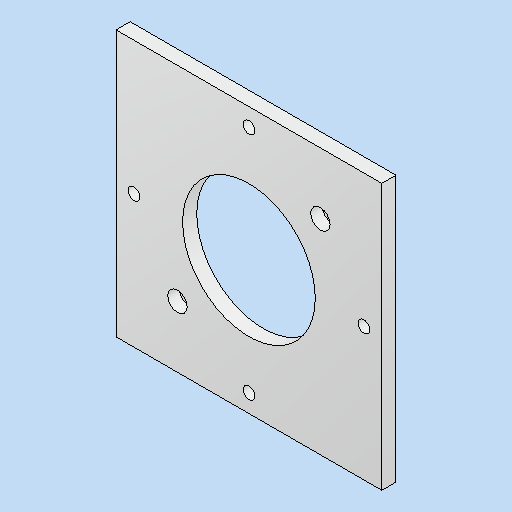
# Autodesk Inventor part: FLI-Al-Plate
Saved by Autodesk Inventor 2025 (Build 290162000, 162)
## iProperties
Created: 2025-02-17
Part Number: FLI-Al-Plate
Material: Aluminum 6061
Document SubType Name: Modeling
Designer: kuzmin
Density: 2.7 g/cm^3
Appearance: Aluminum - Flat
Author: kuzmin
Autodesk Inventor part; units mm, degrees
ref_plane "YZ Plane" through (0, 0, 0) normal (1, 0, 0) x (0, 1, 0)
ref_plane "XZ Plane" through (0, 0, 0) normal (0, 1, 0) x (-1, 0, 0)
ref_plane "XY Plane" through (0, 0, 0) normal (0, 0, 1) x (1, 0, 0)
sketch "Sketch1" plane through (0, 0, 0) normal (0, 0, 1) x (1, 0, 0)
  line L0 (-75.15, 75.15) -> (75.15, 75.15)
  line L1 (75.15, 75.15) -> (75.15, -75.15)
  line L2 (75.15, -75.15) -> (-75.15, -75.15)
  line L3 (-75.15, -75.15) -> (-75.15, 75.15)
  circle A0 centre (40.4112, 40.4112) radius 3.4
  circle A1 centre (-40.4112, -40.4112) radius 3.4
  circle A2 centre (-65, 0) radius 3.35
  circle A3 centre (0, -65) radius 3.35
  circle A4 centre (0, 65) radius 3.35
  circle A5 centre (65, 0) radius 3.35
  circle A6 centre (0, 0) radius 65 construction
  circle A7 centre (0, 0) radius 37.5
  circle A8 centre (0, 0) radius 57.15 construction
  line L4 (40.4112, 40.4112) -> (-40.4112, -40.4112) construction
  point P0 (0, 75.15)
  point P1 (75.15, 0)
  dimension "d14" = 150.3
  dimension "d26" = 6.7
  dimension "d32" = 130
  dimension "d33" = 75
  dimension "d40" = 114.3
  dimension "d42" = 6.8
  dimension "d43" = 45
  constraints: 10 end point, 9 centre point, 6 point on circle, 4 coincident, 4 equal radius, 3 horizontal alignment, 3 midpoint, 3 vertical alignment, 2 parallel, 2 perpendicular, 1 horizontal
  measures "d14" distance of L0.start L0.end
  measures "d26" diameter of A4
  measures "d32" diameter of A6
  measures "d33" diameter of A7
  measures "d40" diameter of A8
  measures "d42" diameter of A0
  measures "d43" angle of L2 L4
extrude "Extrusion1" add sketch "Sketch1" along normal blind 8
sketch "Sketch2" plane through (0, 0, 8) normal (0, 0, 1) x (1, 0, 0)
  circle A0 centre (40.4112, 40.4112) radius 3.4 projected
  circle A1 centre (40.4112, 40.4112) radius 5.5
  circle A2 centre (-40.4112, -40.4112) radius 3.4 projected
  circle A3 centre (-40.4112, -40.4112) radius 5.5
  point P0 (0, 0)
  dimension "d46" = 11
  constraints: 2 centre point, 2 coincident, 1 equal radius
  measures "d46" diameter of A1
extrude "Extrusion2" cut sketch "Sketch2" against normal blind 6.6 contours A0 | A1 | A3
body "Solid1"
